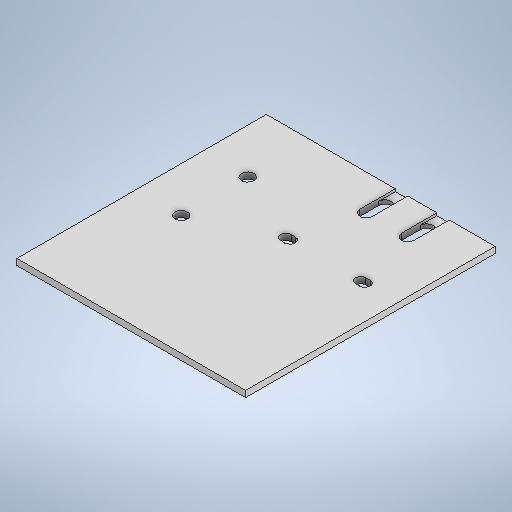
# Autodesk Inventor part: TopMount
Saved by Autodesk Inventor 2025.2 (Build 292293000, 293)
## iProperties
Created: 2025-07-18
Part Number: TopMount
Material: Generic
Document SubType Name: Modeling
Designer: Simon
Density: 1 g/cm^3
Appearance: Default
Author: Simon
Autodesk Inventor part; units mm, degrees
ref_plane "YZ Plane" through (0, 0, 0) normal (1, 0, 0) x (0, 1, 0)
ref_plane "XZ Plane" through (0, 0, 0) normal (0, 1, 0) x (-1, 0, 0)
ref_plane "XY Plane" through (0, 0, 0) normal (0, 0, 1) x (1, 0, 0)
sketch "Sketch1" plane through (0, 0, 0) normal (0, 1, 0) x (-1, 0, 0)
  line L0 (-75, 60) -> (75, 60)
  line L1 (75, 60) -> (75, -60)
  line L2 (75, -60) -> (-75, -60)
  line L3 (-75, -60) -> (-75, 60)
  line L4 (-75, 60) -> (75, -60) construction
  line L5 (75, 60) -> (-75, -60) construction
  point P0 (0, 0)
  dimension "d0" = 150
  dimension "d1" = 120
  constraints: 12 end point, 2 midpoint, 2 parallel, 1 horizontal, 1 perpendicular
  measures "d0" distance of L1.end L2.end
  measures "d1" distance of L0.end L1.end
extrude "Extrusion1" add sketch "Sketch1" along normal blind 3
sketch "Sketch4" plane through (0, 3, 0) normal (0, 1, 0) x (1, 0, 0)
  line L0 (75, 60) -> (-75, 60) projected
  line L1 (-10, 60) -> (10, 60)
  line L2 (10, 60) -> (10, 40)
  line L3 (-10, 60) -> (-10, 40)
  line L4 (-10, 40) -> (10, 40)
  line L5 (-13, 60) -> (-7, 60)
  line L6 (7, 60) -> (13, 60)
  line L7 (-10, 60) -> (-10, 55)
  line L8 (10, 60) -> (10, 55)
  line L9 (-10, 55) -> (-10, 52)
  line L10 (10, 55) -> (10, 52)
  line L11 (-10, 40) -> (-10, 43)
  line L12 (10, 40) -> (10, 43)
  circle A0 centre (-10, 43) radius 3
  circle A1 centre (10, 43) radius 3
  circle A2 centre (-10, 52) radius 3
  circle A3 centre (10, 52) radius 3
  line L13 (-13, 52) -> (-13, 43)
  line L14 (-7, 52) -> (-7, 43)
  line L15 (7, 52) -> (7, 43)
  line L16 (13, 52) -> (13, 43)
  line L17 (-10, 40) -> (-7, 40)
  line L18 (-7, 40) -> (-7, 60)
  line L19 (-7, 60) -> (-10, 60)
  line L20 (-10, 60) -> (-10, 40)
  line L21 (-10, 60) -> (-13, 60)
  line L22 (-13, 60) -> (-13, 40)
  line L23 (-13, 40) -> (-10, 40)
  line L24 (-10, 40) -> (-10, 60)
  line L25 (10, 40) -> (7, 40)
  line L26 (7, 40) -> (7, 60)
  line L27 (7, 60) -> (10, 60)
  line L28 (10, 60) -> (10, 40)
  line L29 (10, 40) -> (13, 40)
  line L30 (13, 40) -> (13, 60)
  line L31 (13, 60) -> (10, 60)
  line L32 (10, 60) -> (10, 40)
  point P0 (0, 0)
  point P1 (0, 60)
  point P2 (7, 60)
  point P3 (7, 52)
  point P4 (-7, 52)
  point P5 (-7, 60)
  point P6 (-13, 60)
  point P7 (-13, 52)
  dimension "d14" = 20
  dimension "d15" = 20
  dimension "d16" = 6
  dimension "d17" = 6
  dimension "d18" = 5
  dimension "d19" = 5
  dimension "d20" = 3
  dimension "d21" = 3
  dimension "d22" = 3
  dimension "d23" = 3
  constraints: 64 end point, 12 point on circle, 10 point on line, 8 parallel, 8 tangent, 6 perpendicular, 4 centre point, 4 coincident, 4 horizontal, 4 midpoint, 1 vertical
  measures "d14" distance of L1.start L1.end
  measures "d15" distance of L1.end L2.end
  measures "d16" distance of L5.start L5.end
  measures "d17" distance of L6.start L6.end
  measures "d18" distance of L1.start L7.end
  measures "d19" distance of L1.end L8.end
  measures "d20" distance of L7.end L9.end
  measures "d21" distance of L8.end L10.end
  measures "d22" distance of L3.end L11.end
  measures "d23" distance of L2.end L12.end
extrude "Extrusion3" cut sketch "Sketch4" against normal through all contours A3 L2 | L16 A1 L2 A3 | L2 A3 | L2 A1 L15 A3 | A1 L2 | L2 A1 | A2 L3 | L14 A0 L3 A2 | L3 A2 | L3 A0 L13 A2 | A0 L3 | L3 A0
extrude "Extrusion5" cut sketch "Sketch4" against normal blind 1.2 contours L30 A3 L2 L0 | L2 A3 L26 L0 | L18 A2 L3 L0 | L3 A2 L22 L0
sketch "Sketch6" plane through (0, 3, 0) normal (0, 1, 0) x (1, 0, 0)
  line L0 (75, 60) -> (-75, 60) projected
  line L1 (0, 60) -> (0, 35)
  line L2 (0, 35) -> (0, -8.2)
  line L3 (0, -8.2) -> (0, 13.4)
  line L4 (0, 13.4) -> (-53.4, 13.4)
  line L5 (-53.4, -2.6) -> (-53.4, 29.4)
  circle A0 centre (-53.4, 29.4) radius 3
  circle A1 centre (-53.4, -2.6) radius 3
  line L6 (-19, 13.4) -> (19, 13.4)
  circle A2 centre (19, 13.4) radius 2.5
  circle A3 centre (-19, 13.4) radius 2.5
  line L7 (-19, 13.4) -> (-17, 13.4)
  line L8 (19, 13.4) -> (17, 13.4)
  circle A4 centre (17, 13.4) radius 2.5
  circle A5 centre (-17, 13.4) radius 2.5
  line L9 (-19, 15.9) -> (-17, 15.9)
  line L10 (-19, 10.9) -> (-17, 10.9)
  line L11 (17, 15.9) -> (19, 15.9)
  line L12 (17, 10.9) -> (19, 10.9)
  point P0 (0, 0)
  dimension "d40" = 25
  dimension "d41" = 43.2
  dimension "d42" = 53.4
  dimension "d43" = 32
  dimension "d44" = 6
  dimension "d45" = 6
  dimension "d46" = 38
  dimension "d47" = 5
  dimension "d48" = 5
  dimension "d49" = 2
  dimension "d50" = 2
  dimension "d51" = 5
  dimension "d52" = 5
  constraints: 24 end point, 8 point on circle, 8 tangent, 6 centre point, 6 coincident, 4 midpoint, 3 point on line, 2 vertical, 1 horizontal, 1 perpendicular
  measures "d40" distance of L1.start L1.end
  measures "d41" distance of L1.end L2.end
  measures "d42" distance of L3.end L4.end
  measures "d43" distance of L5.start L5.end
  measures "d44" diameter of A0
  measures "d45" diameter of A1
  measures "d46" distance of L6.start L6.end
  measures "d47" diameter of A2
  measures "d48" diameter of A3
  measures "d49" distance of L7.start L7.end
  measures "d50" distance of L8.start L8.end
  measures "d51" diameter of A4
  measures "d52" diameter of A5
extrude "Extrusion6" cut sketch "Sketch6" against normal through all
sketch "Sketch7" plane through (0, 3, 0) normal (0, 1, 0) x (1, 0, 0)
  line L0 (75, 60) -> (-75, 60) projected
  line L1 (-75, -60) -> (75, -60) projected
  line L2 (75, 60) -> (35, 60)
  line L3 (35, 60) -> (35, -60)
  line L4 (35, -60) -> (75, -60)
  line L5 (75, -60) -> (75, 60)
  point P0 (0, 0)
  dimension "d55" = 40
  constraints: 8 end point, 2 parallel, 1 horizontal, 1 perpendicular, 1 point on line
  measures "d55" distance of L4.end L3.end
extrude "Extrusion7" cut sketch "Sketch7" against normal through all
body "Solid1"
